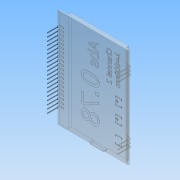
# Autodesk Inventor part: LCD12864-large
Saved by Autodesk Inventor 2016 (Build 200138000, 138)
## iProperties
Created: 2015-10-21
Part Number: LCD12864-large
Material: Polycarbonate, Clear
Document SubType Name: Modeling
Designer: Openlab
Density: 1.2 g/cm^3
Appearance: Polycarbonate - Clear
Author: Openlab
Autodesk Inventor part; units mm, degrees
(part 1 of 2)
ref_plane "YZ Plane" through (0, 0, 0) normal (1, 0, 0) x (0, 1, 0)
ref_plane "XZ Plane" through (0, 0, 0) normal (0, 1, 0) x (-1, 0, 0)
ref_plane "XY Plane" through (0, 0, 0) normal (0, 0, 1) x (1, 0, 0)
sketch "Sketch1" plane through (0, 0, 0) normal (0, 1, 0) x (-1, 0, 0)
  line L0 (-24.25, 34.35) -> (24.25, 34.35)
  line L1 (24.25, 34.35) -> (24.25, -34.35)
  line L2 (24.25, -34.35) -> (-24.25, -34.35)
  line L3 (-24.25, -34.35) -> (-24.25, 34.35)
  line L4 (-24.25, 34.35) -> (24.25, -34.35) construction
  line L5 (24.25, 34.35) -> (-24.25, -34.35) construction
  line L6 (9.9499, 0) -> (-13.7816, 0) construction
  point P0 (0, 0)
  dimension "d0" = 68.7
  dimension "d1" = 48.5
  constraints: 14 end point, 2 horizontal, 2 midpoint, 2 parallel, 1 perpendicular
  measures "d0" distance of L2.end L0.start
  measures "d1" distance of L1.end L2.end
extrude "Extrusion1" add sketch "Sketch1" along normal blind 1.1
sketch "Sketch2" plane through (0, 1.1, 0) normal (0, 1, 0) x (1, 0, 0)
  line L0 (-24.25, -34.35) -> (24.25, -34.35) projected
  line L1 (-24.25, 34.35) -> (-24.25, -34.35) projected
  line L2 (-18.15, -34.35) -> (21.75, -34.35)
  line L3 (21.75, -34.35) -> (21.75, 34.35)
  line L4 (21.75, 34.35) -> (-18.15, 34.35)
  line L5 (-18.15, 34.35) -> (-18.15, -34.35)
  line L6 (24.25, -34.35) -> (24.25, 34.35) projected
  line L7 (-9.9499, 0) -> (13.7816, 0) construction
  line L8 (-24.25, -34.35) -> (24.25, -34.35) projected
  line L9 (24.25, -34.35) -> (24.25, 34.35) projected
  line L10 (24.25, 34.35) -> (-24.25, 34.35) projected
  line L11 (-24.25, 34.35) -> (-24.25, -34.35) projected
  point P0 (0, 0)
  dimension "d4" = 39.9
  dimension "d5" = 2.5
  dimension "d6" = 68.7
  constraints: 8 end point, 2 parallel, 1 horizontal, 1 perpendicular, 1 other
  measures "d4" distance of L2.start L2.end
  measures "d5" distance between parallel lines of L6 L3
  measures "d6" distance between parallel lines of L4 L2
extrude "Extrusion2" add sketch "Sketch2" along normal blind 1.9 contours L5 L4 L3 L0
sketch "Sketch4" plane through (24.25, 0, -34.35) normal (0, 0, -1) x (-1, 0, 0)
  line L0 (25.9, 3) -> (17.9, 3)
  line L1 (16.9, 2) -> (16.9, 1)
  line L2 (17.9, 0) -> (25.9, 0)
  line L3 (26.9, 1) -> (26.9, 2)
  line L4 (48.5, 0) -> (0, 0) projected
  line L5 (2.5, 3) -> (42.4, 3) projected
  arc A0 (17.9, 3) -> (16.9, 2) centre (17.9, 2) ccw
  arc A1 (26.9, 2) -> (25.9, 3) centre (25.9, 2) ccw
  arc A2 (25.9, 0) -> (26.9, 1) centre (25.9, 1) ccw
  arc A3 (16.9, 1) -> (17.9, 0) centre (17.9, 1) ccw
  line L6 (0, 0) -> (0, 1.1) projected
  point P0 (24.25, 0)
  point P1 (16.9, 3)
  point P2 (26.9, 0)
  dimension "d9" = 1
  dimension "d10" = 10
  dimension "d11" = 16.9
  constraints: 8 end point, 8 point on circle, 8 tangent, 6 point on line, 4 centre point, 3 equal radius, 2 parallel, 1 horizontal, 1 perpendicular
  measures "d9" radius of A0
  measures "d10" distance between parallel lines of L1 L3
  measures "d11" distance between parallel lines of L6 L1
extrude "Extrusion3" add sketch "Sketch4" along normal blind 1
fillet "Fillet1" radius 0.5 14 edges at (-2.3571, 0.2929, -34.35) (-2.3571, 2.7071, -34.35) (-2.65, 1.5, -34.35) (7.35, 1.5, -34.35) (7.0571, 0.2929, -34.35) (7.0571, 2.7071, -34.35) (2.35, 3, -35.35) (7.0571, 2.7071, -35.35) (7.35, 1.5, -35.35) (7.0571, 0.2929, -35.35) (2.35, 0, -35.35) (-2.3571, 0.2929, -35.35) (-2.65, 1.5, -35.35) (-2.3571, 2.7071, -35.35)
sketch "Sketch5" plane through (0, 1.1, 0) normal (0, 1, 0) x (1, 0, 0)
  line L0 (-24.25, -24.63) -> (-21.75, -24.63)
  line L1 (-21.75, -24.63) -> (-21.75, -23.63)
  line L2 (-21.75, -23.63) -> (-24.25, -23.63)
  line L3 (-24.25, -23.63) -> (-24.25, -24.63)
  line L4 (-24.25, 34.35) -> (-24.25, -34.35) projected
  line L5 (-24.25, -21.09) -> (-24.25, -22.09)
  line L6 (-21.75, -21.09) -> (-24.25, -21.09)
  line L7 (-21.75, -22.09) -> (-21.75, -21.09)
  line L8 (-24.25, -22.09) -> (-21.75, -22.09)
  line L9 (-24.25, -18.55) -> (-24.25, -19.55)
  line L10 (-21.75, -18.55) -> (-24.25, -18.55)
  line L11 (-21.75, -19.55) -> (-21.75, -18.55)
  line L12 (-24.25, -19.55) -> (-21.75, -19.55)
  line L13 (-24.25, -16.01) -> (-24.25, -17.01)
  line L14 (-21.75, -16.01) -> (-24.25, -16.01)
  line L15 (-21.75, -17.01) -> (-21.75, -16.01)
  line L16 (-24.25, -17.01) -> (-21.75, -17.01)
  line L17 (-24.25, -13.47) -> (-24.25, -14.47)
  line L18 (-21.75, -13.47) -> (-24.25, -13.47)
  line L19 (-21.75, -14.47) -> (-21.75, -13.47)
  line L20 (-24.25, -14.47) -> (-21.75, -14.47)
  line L21 (-24.25, -10.93) -> (-24.25, -11.93)
  line L22 (-21.75, -10.93) -> (-24.25, -10.93)
  line L23 (-21.75, -11.93) -> (-21.75, -10.93)
  line L24 (-24.25, -11.93) -> (-21.75, -11.93)
  line L25 (-24.25, -8.39) -> (-24.25, -9.39)
  line L26 (-21.75, -8.39) -> (-24.25, -8.39)
  line L27 (-21.75, -9.39) -> (-21.75, -8.39)
  line L28 (-24.25, -9.39) -> (-21.75, -9.39)
  line L29 (-24.25, -5.85) -> (-24.25, -6.85)
  line L30 (-21.75, -5.85) -> (-24.25, -5.85)
  line L31 (-21.75, -6.85) -> (-21.75, -5.85)
  line L32 (-24.25, -6.85) -> (-21.75, -6.85)
  line L33 (-24.25, -3.31) -> (-24.25, -4.31)
  line L34 (-21.75, -3.31) -> (-24.25, -3.31)
  line L35 (-21.75, -4.31) -> (-21.75, -3.31)
  line L36 (-24.25, -4.31) -> (-21.75, -4.31)
  line L37 (-24.25, -0.77) -> (-24.25, -1.77)
  line L38 (-21.75, -0.77) -> (-24.25, -0.77)
  line L39 (-21.75, -1.77) -> (-21.75, -0.77)
  line L40 (-24.25, -1.77) -> (-21.75, -1.77)
  line L41 (-24.25, 1.77) -> (-24.25, 0.77)
  line L42 (-21.75, 1.77) -> (-24.25, 1.77)
  line L43 (-21.75, 0.77) -> (-21.75, 1.77)
  line L44 (-24.25, 0.77) -> (-21.75, 0.77)
  line L45 (-24.25, 4.31) -> (-24.25, 3.31)
  line L46 (-21.75, 4.31) -> (-24.25, 4.31)
  line L47 (-21.75, 3.31) -> (-21.75, 4.31)
  line L48 (-24.25, 3.31) -> (-21.75, 3.31)
  line L49 (-24.25, 6.85) -> (-24.25, 5.85)
  line L50 (-21.75, 6.85) -> (-24.25, 6.85)
  line L51 (-21.75, 5.85) -> (-21.75, 6.85)
  line L52 (-24.25, 5.85) -> (-21.75, 5.85)
  line L53 (-24.25, 9.39) -> (-24.25, 8.39)
  line L54 (-21.75, 9.39) -> (-24.25, 9.39)
  line L55 (-21.75, 8.39) -> (-21.75, 9.39)
  line L56 (-24.25, 8.39) -> (-21.75, 8.39)
  line L57 (-24.25, 11.93) -> (-24.25, 10.93)
  line L58 (-21.75, 11.93) -> (-24.25, 11.93)
  line L59 (-21.75, 10.93) -> (-21.75, 11.93)
  line L60 (-24.25, 10.93) -> (-21.75, 10.93)
  line L61 (-24.25, 14.47) -> (-24.25, 13.47)
  line L62 (-21.75, 14.47) -> (-24.25, 14.47)
  line L63 (-21.75, 13.47) -> (-21.75, 14.47)
  line L64 (-24.25, 13.47) -> (-21.75, 13.47)
  line L65 (-24.25, 17.01) -> (-24.25, 16.01)
  line L66 (-21.75, 17.01) -> (-24.25, 17.01)
  line L67 (-21.75, 16.01) -> (-21.75, 17.01)
  line L68 (-24.25, 16.01) -> (-21.75, 16.01)
  line L69 (-24.25, 19.55) -> (-24.25, 18.55)
  line L70 (-21.75, 19.55) -> (-24.25, 19.55)
  line L71 (-21.75, 18.55) -> (-21.75, 19.55)
  line L72 (-24.25, 18.55) -> (-21.75, 18.55)
  line L73 (-24.25, 22.09) -> (-24.25, 21.09)
  line L74 (-21.75, 22.09) -> (-24.25, 22.09)
  line L75 (-21.75, 21.09) -> (-21.75, 22.09)
  line L76 (-24.25, 21.09) -> (-21.75, 21.09)
  line L77 (-24.25, 24.63) -> (-24.25, 23.63)
  line L78 (-21.75, 24.63) -> (-24.25, 24.63)
  line L79 (-21.75, 23.63) -> (-21.75, 24.63)
  line L80 (-24.25, 23.63) -> (-21.75, 23.63)
  line L81 (-18.15, -34.35) -> (21.75, -34.35) projected
  line L82 (-2.768, 34.35) -> (-18.15, 34.35) projected
  line L83 (-8.0372, 0) -> (9.0511, 0) construction
  line L84 (-23.3871, -24.13) -> (-20.0759, -24.13) construction
  line L85 (-23.1, 24.13) -> (-19.8377, 24.13) construction
  line L86 (21.75, -24.63) -> (24.25, -24.63)
  line L87 (24.25, -24.63) -> (24.25, -23.63)
  line L88 (24.25, -23.63) -> (21.75, -23.63)
  line L89 (21.75, -23.63) -> (21.75, -24.63)
  line L90 (24.25, -34.35) -> (24.25, 34.35) projected
  line L91 (21.75, -21.09) -> (21.75, -22.09)
  line L92 (21.75, -22.09) -> (24.25, -22.09)
  line L93 (24.25, -21.09) -> (21.75, -21.09)
  line L94 (21.75, -18.55) -> (21.75, -19.55)
  line L95 (21.75, -19.55) -> (24.25, -19.55)
  line L96 (24.25, -18.55) -> (21.75, -18.55)
  line L97 (22.7116, -24.13) -> (23.7521, -24.13) construction
  line L98 (21.75, 23.63) -> (24.25, 23.63)
  line L99 (24.25, 23.63) -> (24.25, 24.63)
  line L100 (24.25, 24.63) -> (21.75, 24.63)
  line L101 (21.75, 24.63) -> (21.75, 23.63)
  line L102 (21.75, 22.08) -> (21.75, 21.08)
  line L103 (21.75, 21.08) -> (24.25, 21.08)
  line L104 (24.25, 21.08) -> (24.25, 22.08)
  line L105 (24.25, 22.08) -> (21.75, 22.08)
  line L106 (21.75, 19.53) -> (21.75, 18.53)
  line L107 (21.75, 18.53) -> (24.25, 18.53)
  line L108 (24.25, 18.53) -> (24.25, 19.53)
  line L109 (24.25, 19.53) -> (21.75, 19.53)
  line L110 (22.1638, 24.13) -> (23.6023, 24.13) construction
  line L111 (24.25, -22.09) -> (24.25, -21.09)
  line L112 (24.25, -19.55) -> (24.25, -18.55)
  point P0 (0, 0)
  dimension "d15" = 1
  dimension "d16" = 2.5
  dimension "d20" = 2.54
  dimension "d25" = 48.26
  dimension "d42" = 2.5
  dimension "d43" = 1
  dimension "d46" = 2.54
  dimension "d51" = 10.22
  dimension "d52" = 2.5
  dimension "d53" = 1
  dimension "d56" = 2.55
  constraints: 218 end point, 8 horizontal, 6 collinear, 6 parallel, 4 perpendicular, 3 vertical, 1 point on line, 185 other
  measures "d15" distance of L2.end L0.start
  measures "d16" distance of L0.start L0.end
  measures "d20" distance of L2.end L5.start
  measures "d25" distance between parallel lines of L85 L84
  measures "d42" distance of L86.start L86.end
  measures "d43" distance of L88.end L86.start
  measures "d46" distance of L88.end L91.start
  measures "d51" distance between parallel lines of L97 L81
  measures "d52" distance of L98.start L98.end
  measures "d53" distance of L100.end L98.start
  measures "d56" distance of L98.start L102.end
extrude "Extrusion5" add sketch "Sketch5" along normal blind 0.3
sketch "Sketch6" plane through (-24.25, 0, -34.35) normal (-1, 0, 0) x (0, 0, 1)
  line L0 (57.98, -0.1) -> (57.98, 1.4)
  line L1 (57.98, 1.4) -> (58.98, 1.4)
  line L2 (58.98, 1.4) -> (58.98, -0.1)
  line L3 (58.73, -0.25) -> (58.73, -7.1)
  line L4 (58.23, -7.1) -> (58.23, -0.25)
  line L5 (58.58, -7.25) -> (58.38, -7.25)
  line L6 (58.83, -0.25) -> (58.73, -0.25)
  line L7 (58.23, -0.25) -> (58.13, -0.25)
  arc A0 (58.83, -0.25) -> (58.98, -0.1) centre (58.83, -0.1) ccw
  arc A1 (57.98, -0.1) -> (58.13, -0.25) centre (58.13, -0.1) ccw
  arc A2 (58.58, -7.25) -> (58.73, -7.1) centre (58.58, -7.1) ccw
  arc A3 (58.23, -7.1) -> (58.38, -7.25) centre (58.38, -7.1) ccw
  line L8 (58.48, -2.8237) -> (58.48, -4.368) construction
  line L9 (55.94, -2.8237) -> (55.94, -4.368) construction
  line L10 (56.29, -0.25) -> (56.19, -0.25)
  line L11 (55.69, -7.1) -> (55.69, -0.25)
  line L12 (55.69, -0.25) -> (55.59, -0.25)
  arc A4 (56.29, -0.25) -> (56.44, -0.1) centre (56.29, -0.1) ccw
  arc A5 (55.44, -0.1) -> (55.59, -0.25) centre (55.59, -0.1) ccw
  line L13 (55.44, -0.1) -> (55.44, 1.4)
  line L14 (55.44, 1.4) -> (56.44, 1.4)
  line L15 (56.44, 1.4) -> (56.44, -0.1)
  line L16 (56.19, -0.25) -> (56.19, -7.1)
  arc A6 (55.69, -7.1) -> (55.84, -7.25) centre (55.84, -7.1) ccw
  line L17 (56.04, -7.25) -> (55.84, -7.25)
  arc A7 (56.04, -7.25) -> (56.19, -7.1) centre (56.04, -7.1) ccw
  line L18 (53.4, -2.8237) -> (53.4, -4.368) construction
  line L19 (53.75, -0.25) -> (53.65, -0.25)
  line L20 (53.15, -7.1) -> (53.15, -0.25)
  line L21 (53.15, -0.25) -> (53.05, -0.25)
  arc A8 (53.75, -0.25) -> (53.9, -0.1) centre (53.75, -0.1) ccw
  arc A9 (52.9, -0.1) -> (53.05, -0.25) centre (53.05, -0.1) ccw
  line L22 (52.9, -0.1) -> (52.9, 1.4)
  line L23 (52.9, 1.4) -> (53.9, 1.4)
  line L24 (53.9, 1.4) -> (53.9, -0.1)
  line L25 (53.65, -0.25) -> (53.65, -7.1)
  arc A10 (53.15, -7.1) -> (53.3, -7.25) centre (53.3, -7.1) ccw
  line L26 (53.5, -7.25) -> (53.3, -7.25)
  arc A11 (53.5, -7.25) -> (53.65, -7.1) centre (53.5, -7.1) ccw
  line L27 (50.86, -2.8237) -> (50.86, -4.368) construction
  line L28 (51.21, -0.25) -> (51.11, -0.25)
  line L29 (50.61, -7.1) -> (50.61, -0.25)
  line L30 (50.61, -0.25) -> (50.51, -0.25)
  arc A12 (51.21, -0.25) -> (51.36, -0.1) centre (51.21, -0.1) ccw
  arc A13 (50.36, -0.1) -> (50.51, -0.25) centre (50.51, -0.1) ccw
  line L31 (50.36, -0.1) -> (50.36, 1.4)
  line L32 (50.36, 1.4) -> (51.36, 1.4)
  line L33 (51.36, 1.4) -> (51.36, -0.1)
  line L34 (51.11, -0.25) -> (51.11, -7.1)
  arc A14 (50.61, -7.1) -> (50.76, -7.25) centre (50.76, -7.1) ccw
  line L35 (50.96, -7.25) -> (50.76, -7.25)
  arc A15 (50.96, -7.25) -> (51.11, -7.1) centre (50.96, -7.1) ccw
  line L36 (48.32, -2.8237) -> (48.32, -4.368) construction
  line L37 (48.67, -0.25) -> (48.57, -0.25)
  line L38 (48.07, -7.1) -> (48.07, -0.25)
  line L39 (48.07, -0.25) -> (47.97, -0.25)
  arc A16 (48.67, -0.25) -> (48.82, -0.1) centre (48.67, -0.1) ccw
  arc A17 (47.82, -0.1) -> (47.97, -0.25) centre (47.97, -0.1) ccw
  line L40 (47.82, -0.1) -> (47.82, 1.4)
  line L41 (47.82, 1.4) -> (48.82, 1.4)
  line L42 (48.82, 1.4) -> (48.82, -0.1)
  line L43 (48.57, -0.25) -> (48.57, -7.1)
  arc A18 (48.07, -7.1) -> (48.22, -7.25) centre (48.22, -7.1) ccw
  line L44 (48.42, -7.25) -> (48.22, -7.25)
  arc A19 (48.42, -7.25) -> (48.57, -7.1) centre (48.42, -7.1) ccw
  line L45 (45.78, -2.8237) -> (45.78, -4.368) construction
  line L46 (46.13, -0.25) -> (46.03, -0.25)
  line L47 (45.53, -7.1) -> (45.53, -0.25)
  line L48 (45.53, -0.25) -> (45.43, -0.25)
  arc A20 (46.13, -0.25) -> (46.28, -0.1) centre (46.13, -0.1) ccw
  arc A21 (45.28, -0.1) -> (45.43, -0.25) centre (45.43, -0.1) ccw
  line L49 (45.28, -0.1) -> (45.28, 1.4)
  line L50 (45.28, 1.4) -> (46.28, 1.4)
  line L51 (46.28, 1.4) -> (46.28, -0.1)
  line L52 (46.03, -0.25) -> (46.03, -7.1)
  arc A22 (45.53, -7.1) -> (45.68, -7.25) centre (45.68, -7.1) ccw
  line L53 (45.88, -7.25) -> (45.68, -7.25)
  arc A23 (45.88, -7.25) -> (46.03, -7.1) centre (45.88, -7.1) ccw
  line L54 (43.24, -2.8237) -> (43.24, -4.368) construction
  line L55 (43.59, -0.25) -> (43.49, -0.25)
  line L56 (42.99, -7.1) -> (42.99, -0.25)
  line L57 (42.99, -0.25) -> (42.89, -0.25)
  arc A24 (43.59, -0.25) -> (43.74, -0.1) centre (43.59, -0.1) ccw
  arc A25 (42.74, -0.1) -> (42.89, -0.25) centre (42.89, -0.1) ccw
  line L58 (42.74, -0.1) -> (42.74, 1.4)
  line L59 (42.74, 1.4) -> (43.74, 1.4)
  line L60 (43.74, 1.4) -> (43.74, -0.1)
  line L61 (43.49, -0.25) -> (43.49, -7.1)
  arc A26 (42.99, -7.1) -> (43.14, -7.25) centre (43.14, -7.1) ccw
  line L62 (43.34, -7.25) -> (43.14, -7.25)
  arc A27 (43.34, -7.25) -> (43.49, -7.1) centre (43.34, -7.1) ccw
  line L63 (40.7, -2.8237) -> (40.7, -4.368) construction
  line L64 (41.05, -0.25) -> (40.95, -0.25)
  line L65 (40.45, -7.1) -> (40.45, -0.25)
  line L66 (40.45, -0.25) -> (40.35, -0.25)
  arc A28 (41.05, -0.25) -> (41.2, -0.1) centre (41.05, -0.1) ccw
  arc A29 (40.2, -0.1) -> (40.35, -0.25) centre (40.35, -0.1) ccw
  line L67 (40.2, -0.1) -> (40.2, 1.4)
  line L68 (40.2, 1.4) -> (41.2, 1.4)
  line L69 (41.2, 1.4) -> (41.2, -0.1)
  line L70 (40.95, -0.25) -> (40.95, -7.1)
  arc A30 (40.45, -7.1) -> (40.6, -7.25) centre (40.6, -7.1) ccw
  line L71 (40.8, -7.25) -> (40.6, -7.25)
  arc A31 (40.8, -7.25) -> (40.95, -7.1) centre (40.8, -7.1) ccw
  line L72 (38.16, -2.8237) -> (38.16, -4.368) construction
  line L73 (38.51, -0.25) -> (38.41, -0.25)
  line L74 (37.91, -7.1) -> (37.91, -0.25)
  line L75 (37.91, -0.25) -> (37.81, -0.25)
  arc A32 (38.51, -0.25) -> (38.66, -0.1) centre (38.51, -0.1) ccw
  arc A33 (37.66, -0.1) -> (37.81, -0.25) centre (37.81, -0.1) ccw
  line L76 (37.66, -0.1) -> (37.66, 1.4)
  line L77 (37.66, 1.4) -> (38.66, 1.4)
  line L78 (38.66, 1.4) -> (38.66, -0.1)
  line L79 (38.41, -0.25) -> (38.41, -7.1)
  arc A34 (37.91, -7.1) -> (38.06, -7.25) centre (38.06, -7.1) ccw
  line L80 (38.26, -7.25) -> (38.06, -7.25)
  arc A35 (38.26, -7.25) -> (38.41, -7.1) centre (38.26, -7.1) ccw
  line L81 (35.62, -2.8237) -> (35.62, -4.368) construction
  line L82 (35.97, -0.25) -> (35.87, -0.25)
  line L83 (35.37, -7.1) -> (35.37, -0.25)
  line L84 (35.37, -0.25) -> (35.27, -0.25)
  arc A36 (35.97, -0.25) -> (36.12, -0.1) centre (35.97, -0.1) ccw
  arc A37 (35.12, -0.1) -> (35.27, -0.25) centre (35.27, -0.1) ccw
  line L85 (35.12, -0.1) -> (35.12, 1.4)
  line L86 (35.12, 1.4) -> (36.12, 1.4)
  line L87 (36.12, 1.4) -> (36.12, -0.1)
  line L88 (35.87, -0.25) -> (35.87, -7.1)
  arc A38 (35.37, -7.1) -> (35.52, -7.25) centre (35.52, -7.1) ccw
  line L89 (35.72, -7.25) -> (35.52, -7.25)
  arc A39 (35.72, -7.25) -> (35.87, -7.1) centre (35.72, -7.1) ccw
  line L90 (33.08, -2.8237) -> (33.08, -4.368) construction
  line L91 (33.43, -0.25) -> (33.33, -0.25)
  line L92 (32.83, -7.1) -> (32.83, -0.25)
  line L93 (32.83, -0.25) -> (32.73, -0.25)
  arc A40 (33.43, -0.25) -> (33.58, -0.1) centre (33.43, -0.1) ccw
  arc A41 (32.58, -0.1) -> (32.73, -0.25) centre (32.73, -0.1) ccw
  line L94 (32.58, -0.1) -> (32.58, 1.4)
  line L95 (32.58, 1.4) -> (33.58, 1.4)
  line L96 (33.58, 1.4) -> (33.58, -0.1)
  line L97 (33.33, -0.25) -> (33.33, -7.1)
  arc A42 (32.83, -7.1) -> (32.98, -7.25) centre (32.98, -7.1) ccw
  line L98 (33.18, -7.25) -> (32.98, -7.25)
  arc A43 (33.18, -7.25) -> (33.33, -7.1) centre (33.18, -7.1) ccw
  line L99 (30.54, -2.8237) -> (30.54, -4.368) construction
  line L100 (30.89, -0.25) -> (30.79, -0.25)
  line L101 (30.29, -7.1) -> (30.29, -0.25)
  line L102 (30.29, -0.25) -> (30.19, -0.25)
  arc A44 (30.89, -0.25) -> (31.04, -0.1) centre (30.89, -0.1) ccw
  arc A45 (30.04, -0.1) -> (30.19, -0.25) centre (30.19, -0.1) ccw
  line L103 (30.04, -0.1) -> (30.04, 1.4)
  line L104 (30.04, 1.4) -> (31.04, 1.4)
  line L105 (31.04, 1.4) -> (31.04, -0.1)
  line L106 (30.79, -0.25) -> (30.79, -7.1)
  arc A46 (30.29, -7.1) -> (30.44, -7.25) centre (30.44, -7.1) ccw
  line L107 (30.64, -7.25) -> (30.44, -7.25)
  arc A47 (30.64, -7.25) -> (30.79, -7.1) centre (30.64, -7.1) ccw
  line L108 (28, -2.8237) -> (28, -4.368) construction
  line L109 (28.35, -0.25) -> (28.25, -0.25)
  line L110 (27.75, -7.1) -> (27.75, -0.25)
  line L111 (27.75, -0.25) -> (27.65, -0.25)
  arc A48 (28.35, -0.25) -> (28.5, -0.1) centre (28.35, -0.1) ccw
  arc A49 (27.5, -0.1) -> (27.65, -0.25) centre (27.65, -0.1) ccw
  line L112 (27.5, -0.1) -> (27.5, 1.4)
  line L113 (27.5, 1.4) -> (28.5, 1.4)
  line L114 (28.5, 1.4) -> (28.5, -0.1)
  line L115 (28.25, -0.25) -> (28.25, -7.1)
  arc A50 (27.75, -7.1) -> (27.9, -7.25) centre (27.9, -7.1) ccw
  line L116 (28.1, -7.25) -> (27.9, -7.25)
  arc A51 (28.1, -7.25) -> (28.25, -7.1) centre (28.1, -7.1) ccw
  line L117 (25.46, -2.8237) -> (25.46, -4.368) construction
  line L118 (25.81, -0.25) -> (25.71, -0.25)
  line L119 (25.21, -7.1) -> (25.21, -0.25)
  line L120 (25.21, -0.25) -> (25.11, -0.25)
  arc A52 (25.81, -0.25) -> (25.96, -0.1) centre (25.81, -0.1) ccw
  arc A53 (24.96, -0.1) -> (25.11, -0.25) centre (25.11, -0.1) ccw
  line L121 (24.96, -0.1) -> (24.96, 1.4)
  line L122 (24.96, 1.4) -> (25.96, 1.4)
  line L123 (25.96, 1.4) -> (25.96, -0.1)
  line L124 (25.71, -0.25) -> (25.71, -7.1)
  arc A54 (25.21, -7.1) -> (25.36, -7.25) centre (25.36, -7.1) ccw
  line L125 (25.56, -7.25) -> (25.36, -7.25)
  arc A55 (25.56, -7.25) -> (25.71, -7.1) centre (25.56, -7.1) ccw
  line L126 (22.92, -2.8237) -> (22.92, -4.368) construction
  line L127 (23.27, -0.25) -> (23.17, -0.25)
  line L128 (22.67, -7.1) -> (22.67, -0.25)
  line L129 (22.67, -0.25) -> (22.57, -0.25)
  arc A56 (23.27, -0.25) -> (23.42, -0.1) centre (23.27, -0.1) ccw
  arc A57 (22.42, -0.1) -> (22.57, -0.25) centre (22.57, -0.1) ccw
  line L130 (22.42, -0.1) -> (22.42, 1.4)
  line L131 (22.42, 1.4) -> (23.42, 1.4)
  line L132 (23.42, 1.4) -> (23.42, -0.1)
  line L133 (23.17, -0.25) -> (23.17, -7.1)
  arc A58 (22.67, -7.1) -> (22.82, -7.25) centre (22.82, -7.1) ccw
  line L134 (23.02, -7.25) -> (22.82, -7.25)
  arc A59 (23.02, -7.25) -> (23.17, -7.1) centre (23.02, -7.1) ccw
  line L135 (20.38, -2.8237) -> (20.38, -4.368) construction
  line L136 (20.73, -0.25) -> (20.63, -0.25)
  line L137 (20.13, -7.1) -> (20.13, -0.25)
  line L138 (20.13, -0.25) -> (20.03, -0.25)
  arc A60 (20.73, -0.25) -> (20.88, -0.1) centre (20.73, -0.1) ccw
  arc A61 (19.88, -0.1) -> (20.03, -0.25) centre (20.03, -0.1) ccw
  line L139 (19.88, -0.1) -> (19.88, 1.4)
  line L140 (19.88, 1.4) -> (20.88, 1.4)
  line L141 (20.88, 1.4) -> (20.88, -0.1)
  line L142 (20.63, -0.25) -> (20.63, -7.1)
  arc A62 (20.13, -7.1) -> (20.28, -7.25) centre (20.28, -7.1) ccw
  line L143 (20.48, -7.25) -> (20.28, -7.25)
  arc A63 (20.48, -7.25) -> (20.63, -7.1) centre (20.48, -7.1) ccw
  line L144 (17.84, -2.8237) -> (17.84, -4.368) construction
  line L145 (18.19, -0.25) -> (18.09, -0.25)
  line L146 (17.59, -7.1) -> (17.59, -0.25)
  line L147 (17.59, -0.25) -> (17.49, -0.25)
  arc A64 (18.19, -0.25) -> (18.34, -0.1) centre (18.19, -0.1) ccw
  arc A65 (17.34, -0.1) -> (17.49, -0.25) centre (17.49, -0.1) ccw
  line L148 (17.34, -0.1) -> (17.34, 1.4)
  line L149 (17.34, 1.4) -> (18.34, 1.4)
  line L150 (18.34, 1.4) -> (18.34, -0.1)
  line L151 (18.09, -0.25) -> (18.09, -7.1)
  arc A66 (17.59, -7.1) -> (17.74, -7.25) centre (17.74, -7.1) ccw
  line L152 (17.94, -7.25) -> (17.74, -7.25)
  arc A67 (17.94, -7.25) -> (18.09, -7.1) centre (17.94, -7.1) ccw
  line L153 (15.3, -2.8237) -> (15.3, -4.368) construction
  line L154 (15.65, -0.25) -> (15.55, -0.25)
  line L155 (15.05, -7.1) -> (15.05, -0.25)
  line L156 (15.05, -0.25) -> (14.95, -0.25)
  arc A68 (15.65, -0.25) -> (15.8, -0.1) centre (15.65, -0.1) ccw
  arc A69 (14.8, -0.1) -> (14.95, -0.25) centre (14.95, -0.1) ccw
  line L157 (14.8, -0.1) -> (14.8, 1.4)
  line L158 (14.8, 1.4) -> (15.8, 1.4)
  line L159 (15.8, 1.4) -> (15.8, -0.1)
  line L160 (15.55, -0.25) -> (15.55, -7.1)
  arc A70 (15.05, -7.1) -> (15.2, -7.25) centre (15.2, -7.1) ccw
  line L161 (15.4, -7.25) -> (15.2, -7.25)
  arc A71 (15.4, -7.25) -> (15.55, -7.1) centre (15.4, -7.1) ccw
  line L162 (12.76, -2.8237) -> (12.76, -4.368) construction
  line L163 (13.11, -0.25) -> (13.01, -0.25)
  line L164 (12.51, -7.1) -> (12.51, -0.25)
  line L165 (12.51, -0.25) -> (12.41, -0.25)
  arc A72 (13.11, -0.25) -> (13.26, -0.1) centre (13.11, -0.1) ccw
  arc A73 (12.26, -0.1) -> (12.41, -0.25) centre (12.41, -0.1) ccw
  line L166 (12.26, -0.1) -> (12.26, 1.4)
  line L167 (12.26, 1.4) -> (13.26, 1.4)
  line L168 (13.26, 1.4) -> (13.26, -0.1)
  line L169 (13.01, -0.25) -> (13.01, -7.1)
  arc A74 (12.51, -7.1) -> (12.66, -7.25) centre (12.66, -7.1) ccw
  line L170 (12.86, -7.25) -> (12.66, -7.25)
  arc A75 (12.86, -7.25) -> (13.01, -7.1) centre (12.86, -7.1) ccw
  line L171 (10.22, -2.8237) -> (10.22, -4.368) construction
  line L172 (10.57, -0.25) -> (10.47, -0.25)
  line L173 (9.97, -7.1) -> (9.97, -0.25)
  line L174 (9.97, -0.25) -> (9.87, -0.25)
  arc A76 (10.57, -0.25) -> (10.72, -0.1) centre (10.57, -0.1) ccw
  arc A77 (9.72, -0.1) -> (9.87, -0.25) centre (9.87, -0.1) ccw
  line L175 (9.72, -0.1) -> (9.72, 1.4)
  line L176 (9.72, 1.4) -> (10.72, 1.4)
  line L177 (10.72, 1.4) -> (10.72, -0.1)
  line L178 (10.47, -0.25) -> (10.47, -7.1)
  arc A78 (9.97, -7.1) -> (10.12, -7.25) centre (10.12, -7.1) ccw
  line L179 (10.32, -7.25) -> (10.12, -7.25)
  arc A79 (10.32, -7.25) -> (10.47, -7.1) centre (10.32, -7.1) ccw
  line L180 (57.98, 1.4) -> (58.98, 1.4) projected
  point P0 (34.35, 0)
  dimension "d26" = 0.15
  dimension "d27" = 0.5
  dimension "d28" = 1
  dimension "d29" = 1.5
  dimension "d30" = 7
  dimension "d33" = 2.54
  constraints: 360 end point, 160 point on circle, 80 centre point, 21 coincident, 8 tangent, 5 perpendicular, 3 equal radius, 3 horizontal, 3 parallel, 2 collinear, 2 vertical, 609 other
  measures "d26" radius of A0
  measures "d27" distance between parallel lines of L4 L3
  measures "d28" distance of L0.end L1.end
  measures "d29" distance from line of A1.centre L1
  measures "d30" vertical distance of A2.centre A1.centre
  measures "d33" distance of L8.end L9.end
extrude "Extrusion4" add sketch "Sketch6" along normal blind 0.3
sketch "Sketch7" plane through (24.25, 0, 34.35) normal (1, 0, 0) x (0, 0, -1)
  line L0 (9.72, 1.4) -> (10.72, 1.4) projected
  line L1 (9.72, 1.4) -> (10.72, 1.4) projected
  line L2 (10.72, 1.4) -> (10.72, -0.1)
  line L3 (10.57, -0.25) -> (10.47, -0.25) projected
  line L4 (10.57, -0.25) -> (10.47, -0.25)
  line L5 (10.47, -0.25) -> (10.47, -7.1)
  line L6 (9.97, -7.1) -> (9.97, -0.25) projected
  line L7 (9.97, -7.1) -> (9.97, -0.25)
  line L8 (9.97, -0.25) -> (9.87, -0.25)
  line L9 (9.72, -0.1) -> (9.72, 1.4)
  line L10 (9.72, 1.4) -> (10.72, 1.4)
  line L11 (10.32, -7.25) -> (10.12, -7.25)
  arc A0 (9.97, -7.1) -> (10.12, -7.25) centre (10.12, -7.1) ccw
  arc A1 (10.32, -7.25) -> (10.47, -7.1) centre (10.32, -7.1) ccw
  arc A2 (10.57, -0.25) -> (10.72, -0.1) centre (10.57, -0.1) ccw
  arc A3 (9.72, -0.1) -> (9.87, -0.25) centre (9.87, -0.1) ccw
  line L12 (10.32, -7.25) -> (10.12, -7.25) projected
  line L13 (12.51, -0.25) -> (12.41, -0.25)
  line L14 (13.11, -0.25) -> (13.01, -0.25)
  arc A4 (12.26, -0.1) -> (12.41, -0.25) centre (12.41, -0.1) ccw
  arc A5 (13.11, -0.25) -> (13.26, -0.1) centre (13.11, -0.1) ccw
  line L15 (12.26, -0.1) -> (12.26, 1.4)
  line L16 (12.26, 1.4) -> (13.26, 1.4)
  line L17 (13.26, 1.4) -> (13.26, -0.1)
  line L18 (13.01, -0.25) -> (13.01, -7.1)
  line L19 (12.51, -7.1) -> (12.51, -0.25)
  arc A6 (12.86, -7.25) -> (13.01, -7.1) centre (12.86, -7.1) ccw
  line L20 (12.86, -7.25) -> (12.66, -7.25)
  arc A7 (12.51, -7.1) -> (12.66, -7.25) centre (12.66, -7.1) ccw
  line L21 (15.05, -0.25) -> (14.95, -0.25)
  line L22 (15.65, -0.25) -> (15.55, -0.25)
  arc A8 (14.8, -0.1) -> (14.95, -0.25) centre (14.95, -0.1) ccw
  arc A9 (15.65, -0.25) -> (15.8, -0.1) centre (15.65, -0.1) ccw
  line L23 (14.8, -0.1) -> (14.8, 1.4)
  line L24 (14.8, 1.4) -> (15.8, 1.4)
  line L25 (15.8, 1.4) -> (15.8, -0.1)
  line L26 (15.55, -0.25) -> (15.55, -7.1)
  line L27 (15.05, -7.1) -> (15.05, -0.25)
  arc A10 (15.4, -7.25) -> (15.55, -7.1) centre (15.4, -7.1) ccw
  line L28 (15.4, -7.25) -> (15.2, -7.25)
  arc A11 (15.05, -7.1) -> (15.2, -7.25) centre (15.2, -7.1) ccw
  line L29 (17.59, -0.25) -> (17.49, -0.25)
  line L30 (18.19, -0.25) -> (18.09, -0.25)
  arc A12 (17.34, -0.1) -> (17.49, -0.25) centre (17.49, -0.1) ccw
  arc A13 (18.19, -0.25) -> (18.34, -0.1) centre (18.19, -0.1) ccw
  line L31 (17.34, -0.1) -> (17.34, 1.4)
  line L32 (17.34, 1.4) -> (18.34, 1.4)
  line L33 (18.34, 1.4) -> (18.34, -0.1)
  line L34 (18.09, -0.25) -> (18.09, -7.1)
  line L35 (17.59, -7.1) -> (17.59, -0.25)
  arc A14 (17.94, -7.25) -> (18.09, -7.1) centre (17.94, -7.1) ccw
  line L36 (17.94, -7.25) -> (17.74, -7.25)
  arc A15 (17.59, -7.1) -> (17.74, -7.25) centre (17.74, -7.1) ccw
  line L37 (20.13, -0.25) -> (20.03, -0.25)
  line L38 (20.73, -0.25) -> (20.63, -0.25)
  arc A16 (19.88, -0.1) -> (20.03, -0.25) centre (20.03, -0.1) ccw
  arc A17 (20.73, -0.25) -> (20.88, -0.1) centre (20.73, -0.1) ccw
  line L39 (19.88, -0.1) -> (19.88, 1.4)
  line L40 (19.88, 1.4) -> (20.88, 1.4)
  line L41 (20.88, 1.4) -> (20.88, -0.1)
  line L42 (20.63, -0.25) -> (20.63, -7.1)
  line L43 (20.13, -7.1) -> (20.13, -0.25)
  arc A18 (20.48, -7.25) -> (20.63, -7.1) centre (20.48, -7.1) ccw
  line L44 (20.48, -7.25) -> (20.28, -7.25)
  arc A19 (20.13, -7.1) -> (20.28, -7.25) centre (20.28, -7.1) ccw
  line L45 (22.67, -0.25) -> (22.57, -0.25)
  line L46 (23.27, -0.25) -> (23.17, -0.25)
  arc A20 (22.42, -0.1) -> (22.57, -0.25) centre (22.57, -0.1) ccw
  arc A21 (23.27, -0.25) -> (23.42, -0.1) centre (23.27, -0.1) ccw
  line L47 (22.42, -0.1) -> (22.42, 1.4)
  line L48 (22.42, 1.4) -> (23.42, 1.4)
  line L49 (23.42, 1.4) -> (23.42, -0.1)
  line L50 (23.17, -0.25) -> (23.17, -7.1)
  line L51 (22.67, -7.1) -> (22.67, -0.25)
  arc A22 (23.02, -7.25) -> (23.17, -7.1) centre (23.02, -7.1) ccw
  line L52 (23.02, -7.25) -> (22.82, -7.25)
  arc A23 (22.67, -7.1) -> (22.82, -7.25) centre (22.82, -7.1) ccw
  line L53 (25.21, -0.25) -> (25.11, -0.25)
  line L54 (25.81, -0.25) -> (25.71, -0.25)
  arc A24 (24.96, -0.1) -> (25.11, -0.25) centre (25.11, -0.1) ccw
  arc A25 (25.81, -0.25) -> (25.96, -0.1) centre (25.81, -0.1) ccw
  line L55 (24.96, -0.1) -> (24.96, 1.4)
  line L56 (24.96, 1.4) -> (25.96, 1.4)
  line L57 (25.96, 1.4) -> (25.96, -0.1)
  line L58 (25.71, -0.25) -> (25.71, -7.1)
  line L59 (25.21, -7.1) -> (25.21, -0.25)
  arc A26 (25.56, -7.25) -> (25.71, -7.1) centre (25.56, -7.1) ccw
  line L60 (25.56, -7.25) -> (25.36, -7.25)
  arc A27 (25.21, -7.1) -> (25.36, -7.25) centre (25.36, -7.1) ccw
  line L61 (27.75, -0.25) -> (27.65, -0.25)
  line L62 (28.35, -0.25) -> (28.25, -0.25)
  arc A28 (27.5, -0.1) -> (27.65, -0.25) centre (27.65, -0.1) ccw
  arc A29 (28.35, -0.25) -> (28.5, -0.1) centre (28.35, -0.1) ccw
  line L63 (27.5, -0.1) -> (27.5, 1.4)
  line L64 (27.5, 1.4) -> (28.5, 1.4)
  line L65 (28.5, 1.4) -> (28.5, -0.1)
  line L66 (28.25, -0.25) -> (28.25, -7.1)
  line L67 (27.75, -7.1) -> (27.75, -0.25)
  arc A30 (28.1, -7.25) -> (28.25, -7.1) centre (28.1, -7.1) ccw
  line L68 (28.1, -7.25) -> (27.9, -7.25)
  arc A31 (27.75, -7.1) -> (27.9, -7.25) centre (27.9, -7.1) ccw
  line L69 (30.29, -0.25) -> (30.19, -0.25)
  line L70 (30.89, -0.25) -> (30.79, -0.25)
  arc A32 (30.04, -0.1) -> (30.19, -0.25) centre (30.19, -0.1) ccw
  arc A33 (30.89, -0.25) -> (31.04, -0.1) centre (30.89, -0.1) ccw
  line L71 (30.04, -0.1) -> (30.04, 1.4)
  line L72 (30.04, 1.4) -> (31.04, 1.4)
  line L73 (31.04, 1.4) -> (31.04, -0.1)
  line L74 (30.79, -0.25) -> (30.79, -7.1)
  line L75 (30.29, -7.1) -> (30.29, -0.25)
  arc A34 (30.64, -7.25) -> (30.79, -7.1) centre (30.64, -7.1) ccw
  line L76 (30.64, -7.25) -> (30.44, -7.25)
  arc A35 (30.29, -7.1) -> (30.44, -7.25) centre (30.44, -7.1) ccw
  line L77 (32.83, -0.25) -> (32.73, -0.25)
  line L78 (33.43, -0.25) -> (33.33, -0.25)
  arc A36 (32.58, -0.1) -> (32.73, -0.25) centre (32.73, -0.1) ccw
  arc A37 (33.43, -0.25) -> (33.58, -0.1) centre (33.43, -0.1) ccw
  line L79 (32.58, -0.1) -> (32.58, 1.4)
  line L80 (32.58, 1.4) -> (33.58, 1.4)
  line L81 (33.58, 1.4) -> (33.58, -0.1)
  line L82 (33.33, -0.25) -> (33.33, -7.1)
  line L83 (32.83, -7.1) -> (32.83, -0.25)
  arc A38 (33.18, -7.25) -> (33.33, -7.1) centre (33.18, -7.1) ccw
  line L84 (33.18, -7.25) -> (32.98, -7.25)
  arc A39 (32.83, -7.1) -> (32.98, -7.25) centre (32.98, -7.1) ccw
  line L85 (35.37, -0.25) -> (35.27, -0.25)
  line L86 (35.97, -0.25) -> (35.87, -0.25)
  arc A40 (35.12, -0.1) -> (35.27, -0.25) centre (35.27, -0.1) ccw
  arc A41 (35.97, -0.25) -> (36.12, -0.1) centre (35.97, -0.1) ccw
  line L87 (35.12, -0.1) -> (35.12, 1.4)
  line L88 (35.12, 1.4) -> (36.12, 1.4)
  line L89 (36.12, 1.4) -> (36.12, -0.1)
  line L90 (35.87, -0.25) -> (35.87, -7.1)
  line L91 (35.37, -7.1) -> (35.37, -0.25)
  arc A42 (35.72, -7.25) -> (35.87, -7.1) centre (35.72, -7.1) ccw
  line L92 (35.72, -7.25) -> (35.52, -7.25)
  arc A43 (35.37, -7.1) -> (35.52, -7.25) centre (35.52, -7.1) ccw
  line L93 (37.91, -0.25) -> (37.81, -0.25)
  line L94 (38.51, -0.25) -> (38.41, -0.25)
  arc A44 (37.66, -0.1) -> (37.81, -0.25) centre (37.81, -0.1) ccw
  arc A45 (38.51, -0.25) -> (38.66, -0.1) centre (38.51, -0.1) ccw
  line L95 (37.66, -0.1) -> (37.66, 1.4)
  line L96 (37.66, 1.4) -> (38.66, 1.4)
  line L97 (38.66, 1.4) -> (38.66, -0.1)
  line L98 (38.41, -0.25) -> (38.41, -7.1)
  line L99 (37.91, -7.1) -> (37.91, -0.25)
  arc A46 (38.26, -7.25) -> (38.41, -7.1) centre (38.26, -7.1) ccw
  line L100 (38.26, -7.25) -> (38.06, -7.25)
  arc A47 (37.91, -7.1) -> (38.06, -7.25) centre (38.06, -7.1) ccw
  line L101 (40.45, -0.25) -> (40.35, -0.25)
  line L102 (41.05, -0.25) -> (40.95, -0.25)
  arc A48 (40.2, -0.1) -> (40.35, -0.25) centre (40.35, -0.1) ccw
  arc A49 (41.05, -0.25) -> (41.2, -0.1) centre (41.05, -0.1) ccw
  line L103 (40.2, -0.1) -> (40.2, 1.4)
  line L104 (40.2, 1.4) -> (41.2, 1.4)
  line L105 (41.2, 1.4) -> (41.2, -0.1)
  line L106 (40.95, -0.25) -> (40.95, -7.1)
  line L107 (40.45, -7.1) -> (40.45, -0.25)
  arc A50 (40.8, -7.25) -> (40.95, -7.1) centre (40.8, -7.1) ccw
  line L108 (40.8, -7.25) -> (40.6, -7.25)
  arc A51 (40.45, -7.1) -> (40.6, -7.25) centre (40.6, -7.1) ccw
  line L109 (42.99, -0.25) -> (42.89, -0.25)
  line L110 (43.59, -0.25) -> (43.49, -0.25)
  arc A52 (42.74, -0.1) -> (42.89, -0.25) centre (42.89, -0.1) ccw
  arc A53 (43.59, -0.25) -> (43.74, -0.1) centre (43.59, -0.1) ccw
  line L111 (42.74, -0.1) -> (42.74, 1.4)
  line L112 (42.74, 1.4) -> (43.74, 1.4)
  line L113 (43.74, 1.4) -> (43.74, -0.1)
  line L114 (43.49, -0.25) -> (43.49, -7.1)
  line L115 (42.99, -7.1) -> (42.99, -0.25)
  arc A54 (43.34, -7.25) -> (43.49, -7.1) centre (43.34, -7.1) ccw
  line L116 (43.34, -7.25) -> (43.14, -7.25)
  arc A55 (42.99, -7.1) -> (43.14, -7.25) centre (43.14, -7.1) ccw
  line L117 (45.53, -0.25) -> (45.43, -0.25)
  line L118 (46.13, -0.25) -> (46.03, -0.25)
  arc A56 (45.28, -0.1) -> (45.43, -0.25) centre (45.43, -0.1) ccw
  arc A57 (46.13, -0.25) -> (46.28, -0.1) centre (46.13, -0.1) ccw
  line L119 (45.28, -0.1) -> (45.28, 1.4)
  line L120 (45.28, 1.4) -> (46.28, 1.4)
  line L121 (46.28, 1.4) -> (46.28, -0.1)
  line L122 (46.03, -0.25) -> (46.03, -7.1)
  line L123 (45.53, -7.1) -> (45.53, -0.25)
  arc A58 (45.88, -7.25) -> (46.03, -7.1) centre (45.88, -7.1) ccw
  line L124 (45.88, -7.25) -> (45.68, -7.25)
  arc A59 (45.53, -7.1) -> (45.68, -7.25) centre (45.68, -7.1) ccw
  line L125 (48.07, -0.25) -> (47.97, -0.25)
  line L126 (48.67, -0.25) -> (48.57, -0.25)
  arc A60 (47.82, -0.1) -> (47.97, -0.25) centre (47.97, -0.1) ccw
  arc A61 (48.67, -0.25) -> (48.82, -0.1) centre (48.67, -0.1) ccw
  line L127 (47.82, -0.1) -> (47.82, 1.4)
  line L128 (47.82, 1.4) -> (48.82, 1.4)
  line L129 (48.82, 1.4) -> (48.82, -0.1)
  line L130 (48.57, -0.25) -> (48.57, -7.1)
  line L131 (48.07, -7.1) -> (48.07, -0.25)
  arc A62 (48.42, -7.25) -> (48.57, -7.1) centre (48.42, -7.1) ccw
  line L132 (48.42, -7.25) -> (48.22, -7.25)
  arc A63 (48.07, -7.1) -> (48.22, -7.25) centre (48.22, -7.1) ccw
  line L133 (50.61, -0.25) -> (50.51, -0.25)
  line L134 (51.21, -0.25) -> (51.11, -0.25)
  arc A64 (50.36, -0.1) -> (50.51, -0.25) centre (50.51, -0.1) ccw
  arc A65 (51.21, -0.25) -> (51.36, -0.1) centre (51.21, -0.1) ccw
  line L135 (50.36, -0.1) -> (50.36, 1.4)
  line L136 (50.36, 1.4) -> (51.36, 1.4)
  line L137 (51.36, 1.4) -> (51.36, -0.1)
  line L138 (51.11, -0.25) -> (51.11, -7.1)
  line L139 (50.61, -7.1) -> (50.61, -0.25)
  arc A66 (50.96, -7.25) -> (51.11, -7.1) centre (50.96, -7.1) ccw
  line L140 (50.96, -7.25) -> (50.76, -7.25)
  arc A67 (50.61, -7.1) -> (50.76, -7.25) centre (50.76, -7.1) ccw
  line L141 (53.15, -0.25) -> (53.05, -0.25)
  line L142 (53.75, -0.25) -> (53.65, -0.25)
  arc A68 (52.9, -0.1) -> (53.05, -0.25) centre (53.05, -0.1) ccw
  arc A69 (53.75, -0.25) -> (53.9, -0.1) centre (53.75, -0.1) ccw
  line L143 (52.9, -0.1) -> (52.9, 1.4)
  line L144 (52.9, 1.4) -> (53.9, 1.4)
  line L145 (53.9, 1.4) -> (53.9, -0.1)
  line L146 (53.65, -0.25) -> (53.65, -7.1)
  line L147 (53.15, -7.1) -> (53.15, -0.25)
  arc A70 (53.5, -7.25) -> (53.65, -7.1) centre (53.5, -7.1) ccw
  line L148 (53.5, -7.25) -> (53.3, -7.25)
  arc A71 (53.15, -7.1) -> (53.3, -7.25) centre (53.3, -7.1) ccw
  line L149 (55.69, -0.25) -> (55.59, -0.25)
  line L150 (56.29, -0.25) -> (56.19, -0.25)
  arc A72 (55.44, -0.1) -> (55.59, -0.25) centre (55.59, -0.1) ccw
  arc A73 (56.29, -0.25) -> (56.44, -0.1) centre (56.29, -0.1) ccw
  line L151 (55.44, -0.1) -> (55.44, 1.4)
  line L152 (55.44, 1.4) -> (56.44, 1.4)
  line L153 (56.44, 1.4) -> (56.44, -0.1)
  line L154 (56.19, -0.25) -> (56.19, -7.1)
  line L155 (55.69, -7.1) -> (55.69, -0.25)
  arc A74 (56.04, -7.25) -> (56.19, -7.1) centre (56.04, -7.1) ccw
  line L156 (56.04, -7.25) -> (55.84, -7.25)
  arc A75 (55.69, -7.1) -> (55.84, -7.25) centre (55.84, -7.1) ccw
  line L157 (58.23, -0.25) -> (58.13, -0.25)
  line L158 (58.83, -0.25) -> (58.73, -0.25)
  arc A76 (57.98, -0.1) -> (58.13, -0.25) centre (58.13, -0.1) ccw
  arc A77 (58.83, -0.25) -> (58.98, -0.1) centre (58.83, -0.1) ccw
  line L159 (57.98, -0.1) -> (57.98, 1.4)
  line L160 (57.98, 1.4) -> (58.98, 1.4)
  line L161 (58.98, 1.4) -> (58.98, -0.1)
  line L162 (58.73, -0.25) -> (58.73, -7.1)
  line L163 (58.23, -7.1) -> (58.23, -0.25)
  arc A78 (58.58, -7.25) -> (58.73, -7.1) centre (58.58, -7.1) ccw
  line L164 (58.58, -7.25) -> (58.38, -7.25)
  arc A79 (58.23, -7.1) -> (58.38, -7.25) centre (58.38, -7.1) ccw
  point P0 (34.35, 0)
  point P1 (9.72, -0.25)
  point P2 (12.26, -0.25)
  point P3 (13.11, -0.25)
  point P4 (12.86, -7.25)
  point P5 (12.66, -7.25)
  point P6 (14.8, -0.25)
  point P7 (15.65, -0.25)
  point P8 (15.4, -7.25)
  point P9 (15.2, -7.25)
  point P10 (17.34, -0.25)
  point P11 (18.19, -0.25)
  point P12 (17.94, -7.25)
  point P13 (17.74, -7.25)
  point P14 (19.88, -0.25)
  point P15 (20.73, -0.25)
  point P16 (20.48, -7.25)
  point P17 (20.28, -7.25)
  point P18 (22.42, -0.25)
  point P19 (23.27, -0.25)
  point P20 (23.02, -7.25)
  point P21 (22.82, -7.25)
  point P22 (24.96, -0.25)
  point P23 (25.81, -0.25)
  point P24 (25.56, -7.25)
  point P25 (25.36, -7.25)
  point P26 (27.5, -0.25)
  point P27 (28.35, -0.25)
  point P28 (28.1, -7.25)
  point P29 (27.9, -7.25)
  point P30 (30.04, -0.25)
  point P31 (30.89, -0.25)
  point P32 (30.64, -7.25)
  point P33 (30.44, -7.25)
  point P34 (32.58, -0.25)
  point P35 (33.43, -0.25)
  point P36 (33.18, -7.25)
  point P37 (32.98, -7.25)
  point P38 (35.12, -0.25)
  point P39 (35.97, -0.25)
  point P40 (35.72, -7.25)
  point P41 (35.52, -7.25)
  point P42 (37.66, -0.25)
  point P43 (38.51, -0.25)
  point P44 (38.26, -7.25)
  point P45 (38.06, -7.25)
  point P46 (40.2, -0.25)
  point P47 (41.05, -0.25)
  point P48 (40.8, -7.25)
  point P49 (40.6, -7.25)
  point P50 (42.74, -0.25)
  point P51 (43.59, -0.25)
  point P52 (43.34, -7.25)
  point P53 (43.14, -7.25)
  point P54 (45.28, -0.25)
  point P55 (46.13, -0.25)
  point P56 (45.88, -7.25)
  point P57 (45.68, -7.25)
  point P58 (47.82, -0.25)
  point P59 (48.67, -0.25)
  point P60 (48.42, -7.25)
  point P61 (48.22, -7.25)
  point P62 (50.36, -0.25)
  point P63 (51.21, -0.25)
  point P64 (50.96, -7.25)
  point P65 (50.76, -7.25)
  point P66 (52.9, -0.25)
  point P67 (53.75, -0.25)
  point P68 (53.5, -7.25)
  point P69 (53.3, -7.25)
  point P70 (55.44, -0.25)
  point P71 (56.29, -0.25)
  point P72 (56.04, -7.25)
  point P73 (55.84, -7.25)
  point P74 (57.98, -0.25)
  point P75 (58.83, -0.25)
  point P76 (58.58, -7.25)
  point P77 (58.38, -7.25)
  dimension "d61" = 0.15
  dimension "d64" = 2.54
  constraints: 320 end point, 160 point on circle, 80 centre point, 60 point on line, 8 tangent, 3 collinear, 3 equal radius, 3 perpendicular, 2 horizontal, 1 vertical, 627 other
  measures "d61" radius of A0
  measures "d64" distance of L0.start L15.end
extrude "Extrusion6" add sketch "Sketch7" along normal blind 0.3 contours L0 L2 A2 L3 L5 A1 L11 A0 L6 L8 A3 L9 | L13 A4 L15 L16 L17 A5 L14 L18 A6 L20 A7 L19 | L21 A8 L23 L24 L25 A9 L22 L26 A10 L28 A11 L27 | L141 A68 L143 L144 L145 A69 L142 L146 A70 L148 A71 L147 | L149 A72 L151 L152 L153 A73 L150 L154 A74 L156 A75 L155 | L157 A76 L159 L160 L161 A77 L158 L162 A78 L164 A79 L163